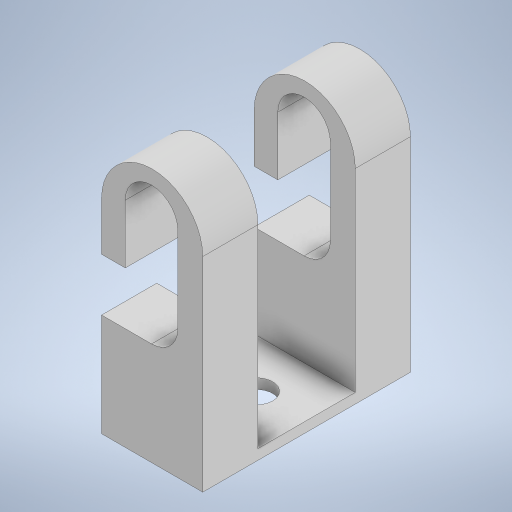
# Autodesk Inventor part: 6 Backet Adjustment
Saved by Autodesk Inventor 2024 (Build 280153000, 153)
## iProperties
Created: 2023-10-21
Part Number: 6 Backet Adjustment
Material: Generic
Document SubType Name: Modeling
Designer: olson
Density: 1 g/cm^3
Appearance: Default
Author: olson
Autodesk Inventor part; units mm, degrees
ref_plane "YZ Plane" through (0, 0, 0) normal (1, 0, 0) x (0, 1, 0)
ref_plane "XZ Plane" through (0, 0, 0) normal (0, 1, 0) x (-1, 0, 0)
ref_plane "XY Plane" through (0, 0, 0) normal (0, 0, 1) x (1, 0, 0)
sketch "Sketch1" plane through (0, 0, 0) normal (0, 1, 0) x (-1, 0, 0)
  line L0 (10, 31.05) -> (-10, 31.05)
  line L1 (-10, 31.05) -> (-10, -10)
  line L2 (-10, -10) -> (10, -10)
  line L3 (10, -10) -> (10, 31.05)
  point P0 (0, 0)
  dimension "d0" = 20
  dimension "d1" = 41.05
  constraints: 8 end point, 2 parallel, 1 horizontal, 1 perpendicular
  measures "d0" distance of L2.end L1.end
  measures "d1" distance of L1.end L0.end
extrude "Extrusion1" add sketch "Sketch1" along normal blind 2
sketch "Sketch2" plane through (0, 2, 0) normal (0, 1, 0) x (1, 0, 0)
  line L0 (-10, -31.05) -> (10, -31.05) projected
  line L1 (0, -31.05) -> (-6.35, -31.05)
  line L2 (-6.35, -20.15) -> (6.35, -20.15)
  line L3 (6.35, -31.05) -> (0, -31.05)
  line L4 (10, 10) -> (-10, 10) projected
  line L5 (-6.35, -0.9) -> (6.35, -0.9)
  line L6 (-6.35, 10) -> (6.35, 10)
  line L7 (-6.35, -31.05) -> (-10, -31.05)
  line L8 (-10, 10) -> (-10, -31.05) projected
  line L9 (-10, -20.15) -> (-6.35, -20.15)
  line L10 (6.35, -31.05) -> (10, -31.05)
  line L11 (10, -31.05) -> (10, 10) projected
  line L12 (10, -20.15) -> (6.35, -20.15)
  line L13 (6.35, -0.9) -> (10, -0.9)
  line L14 (10, 10) -> (6.35, 10)
  line L15 (10, -0.9) -> (10, 10)
  line L16 (10, -31.05) -> (10, -20.15)
  line L17 (-10, -31.05) -> (-10, -20.15)
  line L18 (-6.35, -0.9) -> (-10, -0.9)
  line L19 (-10, -0.9) -> (-10, 10)
  line L20 (-10, 10) -> (-6.35, 10)
  point P0 (0, 0)
  dimension "d4" = 6.35
  dimension "d5" = 10.9
  dimension "d6" = 12.7
  dimension "d7" = 10.9
  constraints: 34 end point, 9 point on line, 7 perpendicular, 4 collinear, 1 horizontal, 1 midpoint, 1 parallel, 1 vertical
  measures "d4" distance of L1.start L1.end
  measures "d5" distance of L1.end L2.start
  measures "d6" distance of L2.start L2.end
  measures "d7" distance of L6.start L5.start
extrude "Extrusion2" add sketch "Sketch2" along normal blind 48.3354 contours L8 L9 L2 L12 L11 L0 | L8 L4 L11 L13 L5 L18
sketch "Sketch9" plane through (-10, 0, 31.05) normal (0, 0, 1) x (1, 0, 0)
  arc A0 (15.084, 42.3223) -> (4.684, 42.3223) centre (9.884, 42.3223) ccw
  line L0 (15.084, 35.9247) -> (15.084, 42.3223)
  line L1 (4.684, 41.1247) -> (4.684, 42.3223)
  arc A1 (15.084, 42.3223) -> (4.684, 42.3223) centre (9.884, 42.3223) ccw
  line L2 (4.684, 42.3223) -> (4.684, 35.9247)
  line L3 (9.8827, 20.3222) -> (-0.0013, 20.3222)
  line L4 (-0.0013, 30.726) -> (-0.0013, 20.3222)
  line L5 (4.684, 35.9247) -> (4.684, 30.726)
  line L6 (15.084, 35.9247) -> (15.0853, 25.5254)
  arc A2 (15.084, 35.9247) -> (15.084, 35.9251) centre (9.884, 35.9243) ccw
  line L7 (4.684, 30.726) -> (-0.0013, 30.726)
  arc A3 (9.8827, 20.3222) -> (15.0853, 25.5254) centre (9.8827, 25.5248) ccw
  point P0 (10, 0)
  constraints: 16 end point, 8 point on circle, 4 centre point, 3 tangent, 2 horizontal, 2 perpendicular, 2 point on line, 1 coincident, 1 vertical
fillet "Fillet4" radius 10 4 edges at (10, 50.3354, 25.6) (-10, 50.3354, 25.6) (-10, 50.3354, -4.55) (10, 50.3354, -4.55)
sketch "Sketch10" plane through (0, 2, 0) normal (0, 1, 0) x (1, 0, 0)
  line L0 (10, -31.05) -> (-10, -31.05) projected
  line L1 (-10, 10) -> (10, 10) projected
  line L2 (10, -20.15) -> (10, -0.9) projected
  line L3 (-10, -0.9) -> (-10, -20.15) projected
  line L4 (10, -10.525) -> (-10, -10.525)
  circle A0 centre (0, -10.525) radius 3.302
  point P0 (0, 0)
  dimension "d53" = 41.05
  dimension "d54" = 6.604
  constraints: 3 midpoint, 2 end point, 1 centre point
  measures "d53" distance between parallel lines of L0 L1
  measures "d54" diameter of A0
extrude "Extrusion10" cut sketch "Sketch10" against normal blind 2
extrude "Extrusion11" cut sketch "Sketch9" against normal through all
body "Solid1"
